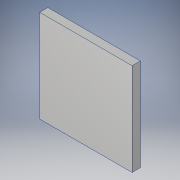
# Autodesk Inventor part: Mounting Plate
Saved by Autodesk Inventor 2019 (Build 230136000, 136)
## iProperties
Created: 2019-08-29
Part Number: Mounting Plate
Material: Aluminum 6061
Document SubType Name: Modeling
Designer: Rick Szalay
Density: 2.7 g/cm^3
Appearance: Aluminum - Flat
Author: Rick Szalay
Autodesk Inventor part; units mm, degrees
ref_plane "YZ Plane" through (0, 0, 0) normal (1, 0, 0) x (0, 1, 0)
ref_plane "XZ Plane" through (0, 0, 0) normal (0, 1, 0) x (-1, 0, 0)
ref_plane "XY Plane" through (0, 0, 0) normal (0, 0, 1) x (1, 0, 0)
sketch "Sketch1" plane through (0, 0, 0) normal (0, 0, 1) x (1, 0, 0)
  line L0 (88.9, -88.9) -> (-88.9, -88.9)
  line L1 (-88.9, -88.9) -> (-88.9, 88.9)
  line L2 (-88.9, 88.9) -> (88.9, 88.9)
  line L3 (88.9, 88.9) -> (88.9, -88.9)
  line L4 (88.9, -88.9) -> (-88.9, 88.9) construction
  line L5 (-88.9, -88.9) -> (88.9, 88.9) construction
  point P0 (0, 0)
  dimension "d2" = 177.8
  constraints: 12 end point, 2 midpoint, 2 parallel, 2 perpendicular, 1 horizontal
  measures "d2" distance of L0.end L1.end
extrude "Extrusion1" add sketch "Sketch1" along normal blind 15.875
body "Solid1"
